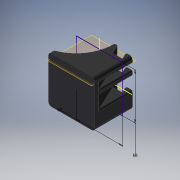
# Autodesk Inventor part: iphonextand-tri
Saved by Autodesk Inventor 2017 (Build 210142000, 142)
## iProperties
Created: 2018-05-22
Part Number: iphonextand-tri
Material: Generic
Document SubType Name: Modeling
Designer: 45027374
Density: 1 g/cm^3
Appearance: Default
Author: 45027374
Autodesk Inventor part; units mm, degrees
ref_plane "YZ Plane" through (0, 0, 0) normal (1, 0, 0) x (0, 1, 0)
ref_plane "XZ Plane" through (0, 0, 0) normal (0, 1, 0) x (-1, 0, 0)
ref_plane "XY Plane" through (0, 0, 0) normal (0, 0, 1) x (1, 0, 0)
sketch "Sketch1" plane through (0, 0, 0) normal (0, 1, 0) x (-1, 0, 0)
  line L0 (30, 30) -> (-30, 30)
  line L1 (-30, 30) -> (-30, -30)
  line L2 (-30, -30) -> (30, -30)
  line L3 (30, -30) -> (30, 30)
  line L4 (42, 0) -> (-42, 0) projected
  line L5 (0, -42) -> (0, 42) projected
  point P0 (0, 0)
  dimension "d0" = 60
  dimension "d1" = 60
  constraints: 8 end point, 2 parallel, 1 horizontal, 1 perpendicular, 2 other
  measures "d0" distance of L0.end L1.end
  measures "d1" distance of L1.end L2.end
extrude "Extrusion1" add sketch "Sketch1" along normal blind 16
sketch "Sketch2" plane through (-30, 0, 30) normal (0, 0, 1) x (1, 0, 0)
  line L0 (0, 16) -> (60, 16) projected
  line L1 (50.4043, 16) -> (56, 4)
  line L2 (56, 4) -> (43.5, 4)
  line L3 (43.5, 4) -> (37.9043, 16)
  line L4 (0, 0) -> (60, 0) projected
  line L5 (60, 0) -> (60, 16) projected
  point P0 (30, 0)
  dimension "d4" = 65
  dimension "d5" = 4
  dimension "d6" = 4
  dimension "d7" = 12.5
  constraints: 6 end point, 2 parallel, 2 point on line
  measures "d4" angle of L1 L0
  measures "d5" distance between parallel lines of L2 L4
  measures "d6" distance from line of L5 L1.end
  measures "d7" distance of L1.end L2.end
extrude "Extrusion2" add sketch "Sketch1" against normal blind 36
extrude "Extrusion3" cut sketch "Sketch2" against normal through all
sketch "Sketch3" plane through (30, 16, 30) normal (1, 0, 0) x (0, 0, -1)
  line L0 (0, 0) -> (60, 0) projected
  line L1 (0, -52) -> (60, -52) projected
  line L2 (22, 0) -> (38, 0)
  line L3 (38, 0) -> (38, -52)
  line L4 (38, -52) -> (22, -52)
  line L5 (22, -52) -> (22, 0)
  line L6 (0, -52) -> (0, 0) projected
  point P0 (30, -16)
  dimension "d12" = 16
  dimension "d13" = 22
  constraints: 8 end point, 2 parallel, 2 point on line, 1 horizontal, 1 perpendicular
  measures "d12" distance between parallel lines of L3 L5
  measures "d13" distance between parallel lines of L6 L5
extrude "Extrusion4" [suppressed]
sketch "Sketch4" plane through (30, -36, 30) normal (1, 0, 0) x (0, 0, -1)
  line L0 (60, 52) -> (0, 52) projected
  line L1 (15.5, 52) -> (8, 52)
  line L2 (8, 52) -> (8, 15)
  line L3 (8, 15) -> (15.5, 15)
  line L4 (15.5, 15) -> (15.5, 52)
  line L5 (22, 0) -> (22, 52) projected
  line L6 (0, 40) -> (60, 40) projected
  point P0 (30, 36)
  point P1 (22, 40)
  dimension "d16" = 6.5
  dimension "d17" = 14
  dimension "d18" = 25
  constraints: 8 end point, 2 parallel, 1 horizontal, 1 perpendicular, 1 point on line
  measures "d16" distance between parallel lines of L4 L5
  measures "d17" distance between parallel lines of L2 L5
  measures "d18" distance between parallel lines of L3 L6
extrude "Extrusion5" [suppressed]
sketch "Sketch5" plane through (-30, -36, 30) normal (0, 0, 1) x (1, 0, 0)
  line L0 (0, 0) -> (0, 52) projected
  line L1 (37.9043, 52) -> (0, 52) projected
  arc A0 (0, 4) -> (33.9043, 52) centre (-14.0496, 49.8978) ccw
  line L2 (0, 52) -> (37.9043, 52) projected
  line L3 (33.9043, 52) -> (0, 52)
  line L4 (0, 52) -> (0, 4)
  point P0 (30, 36)
  dimension "d21" = 4
  dimension "d22" = 4
  dimension "d23" = 48
  constraints: 4 end point, 2 point on circle, 2 point on line, 1 centre point, 1 collinear, 1 perpendicular
  measures "d21" distance of L3.start L1.start
  measures "d22" distance of L4.end L0.start
  measures "d23" radius of A0
extrude "Extrusion6" cut sketch "Sketch5" against normal through all
fillet "Fillet1" radius 3 1 edges at (7.9043, 16, 0)
fillet "Fillet5" [suppressed]
sketch "Sketch8" plane through (0, 16, 0) normal (0, 1, 0) x (1, 0, 0)
  line L0 (20.4043, 30) -> (20.4043, -30) projected
  line L1 (30, -30) -> (-30, -30) projected
  line L2 (20.4043, 30) -> (30, 30)
  line L3 (30, 30) -> (30, -30)
  line L4 (30, -30) -> (20.4043, -30)
  line L5 (20.4043, -30) -> (20.4043, 30)
  point P0 (0, 0)
  point P1 (20.4043, 8)
  point P2 (20.4043, -14.5)
  constraints: 8 end point, 2 parallel, 1 horizontal, 1 perpendicular
extrude "Extrusion7" cut sketch "Sketch8" against normal blind 3
fillet "Fillet6" radius 1.5 1 edges at (21.8032, 13, 0)
fillet "Fillet9" radius 4 4 edges at (30, -11.5, 30) (30, -11.5, -30) (-30, -34, -30) (-30, -34, 30)
fillet "Fillet10" [suppressed]
fillet "Fillet11" radius 2 1 edges at (3.9043, 16, 0)
sketch "Sketch9" plane through (0, 0, 0) normal (0, 0, 1) x (1, 0, 0)
  line L0 (30, 13) -> (30, -36) projected
  line L1 (-50.0912, 0) -> (90.5304, 0) projected
  line L2 (13.5, 4) -> (8.712, 14.2679) projected
  line L3 (7.9043, 16) -> (32.1523, -36)
  line L4 (32.1523, -36) -> (57.1523, -36)
  line L5 (57.1523, -36) -> (32.9043, 16)
  line L6 (57.1523, -36) -> (114.528, -36) construction
  line L7 (32.9043, 16) -> (7.9043, 16)
  point P0 (0, 0)
  dimension "d48" = 115
  dimension "d49" = 36
  dimension "d61" = 25
  dimension "d62" = 16
  constraints: 10 end point, 3 horizontal, 1 collinear, 1 equal length
  measures "d48" angle of L6 L5
  measures "d49" distance between parallel lines of L1 L4
  measures "d61" distance of L3.end L4.end
  measures "d62" distance between parallel lines of L7 L1
extrude "Extrusion8" cut sketch "Sketch9" along normal mid plane 16
fillet "Fillet12" radius 2 2 edges at (30, -9.1922, 8) (30, -9.1922, -8)
ref_plane "Work Plane1" through (-26, -36, 22) normal (0, 0, 1) x (1, 0, 0)
sketch "Sketch10" plane through (-26, -36, 22) normal (0, 0, 1) x (1, 0, 0)
  line L0 (33.9043, 52) -> (58.1523, 0)
  line L1 (34.712, 50.2679) -> (39.5, 40) projected
  line L2 (58.1523, 0) -> (83.1523, 0)
  line L3 (83.1523, 0) -> (58.9043, 52)
  line L4 (58.9043, 52) -> (33.9043, 52)
  line L5 (39.5, 40) -> (34.712, 50.2679) projected
  line L6 (-20.4333, 36) -> (94.5832, 36) projected
  point P0 (26, 36)
  dimension "d54" = 25
  dimension "d55" = 36
  dimension "d56" = 16
  constraints: 8 end point, 2 collinear, 2 parallel, 1 horizontal
  measures "d54" distance of L0.end L2.end
  measures "d55" distance between parallel lines of L6 L2
  measures "d56" distance between parallel lines of L6 L4
extrude "Extrusion9" cut sketch "Sketch10" against normal blind 7.5
fillet "Fillet13" radius 2 2 edges at (30, -9.1922, 22) (30, -9.1922, 14.5)
fillet "Fillet14" radius 1.5 3 edges at (30, -31.3844, 0) (30, -31.3844, 13.5) (30, -31.3844, 23)
body "Solid1"
